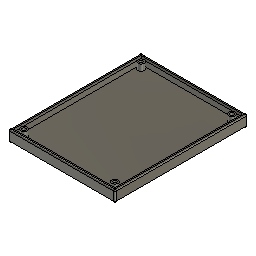
lazyahh_asm (Autodesk Fusion 360 archive; units mm, degrees)
design "ROOM case"
Autodesk Fusion 360 part; units mm, degrees
sketch "Sketch1" plane through (0, 0, 0) normal (0, 0, 1) x (1, 0, 0)
  line L0 (39.5, -50) -> (-39.5, -50)
  line L1 (-39.5, -50) -> (-39.5, 50)
  line L2 (-39.5, 50) -> (39.5, 50)
  line L3 (39.5, 50) -> (39.5, -50)
  line L4 (39.5, -50) -> (-39.5, 50) construction
  line L5 (-39.5, -50) -> (39.5, 50) construction
  line L6 (39.5, 50) -> (36.55, 50)
  line L7 (36.55, 50) -> (36.55, 47.05)
  circle A0 centre (36.55, 47.05) radius 1.35
  circle A1 centre (36.55, 47.05) radius 2.5
  circle A2 centre (36.55, 47.05) radius 2.5
  circle A3 centre (36.55, 47.05) radius 1.35
  line L8 (-39.5, 50) -> (-39.5, 47.05)
  line L9 (-39.5, 47.05) -> (-36.55, 47.05)
  circle A4 centre (36.55, 47.05) radius 1.35
  circle A5 centre (36.55, 47.05) radius 2.5
  circle A6 centre (-36.55, 47.05) radius 1.35
  circle A7 centre (-36.55, 47.05) radius 2.5
  line L10 (0, 0) -> (5, 0)
  circle A8 centre (-36.55, -47.05) radius 2.5
  circle A9 centre (36.55, -47.05) radius 1.35
  circle A10 centre (36.55, -47.05) radius 2.5
  circle A11 centre (-36.55, -47.05) radius 1.35
  line L11 (-42.75, 53.25) -> (42.75, 53.25)
  line L12 (42.75, 53.25) -> (42.75, -53.25)
  line L13 (42.75, -53.25) -> (-42.75, -53.25)
  line L14 (-42.75, -53.25) -> (-42.75, 53.25)
  line L15 (39.75, 50.25) -> (39.75, -50.25)
  line L16 (39.75, -50.25) -> (-39.75, -50.25)
  line L17 (-39.75, -50.25) -> (-39.75, 50.25)
  line L18 (-39.75, 50.25) -> (39.75, 50.25)
  point P0 (36.55, -47.05)
  dimension "d1" = 79
  dimension "d2" = 100
  dimension "d3" = 2.95
  dimension "d4" = 2.95
  dimension "d5" = 2.7
  dimension "d6" = 5
  dimension "d7" = 2.7
  dimension "d8" = 5
  dimension "d9" = 2.95
  dimension "d10" = 2.7
  dimension "d11" = 5
  dimension "d12" = 2.7
  dimension "d13" = 5
  dimension "d14" = -3.25
  dimension "d15" = -0.25
  constraint horizontal L0
  constraint perpendicular L0 L1
  constraint parallel L0 L2
  constraint parallel L1 L3
  constraint coincident L4 L10.start
  constraint coincident L5 L10.start
  constraint coincident L10.start origin
  constraint perpendicular L3 L6
  constraint perpendicular L6 L7
  constraint coincident L7.end A0.centre
  constraint concentric A0 A1
  constraint concentric A2 A3
  constraint perpendicular L2 L8
  constraint perpendicular L1 L9
  constraint coincident L9.end A6.centre
  constraint concentric A6 A7
  constraint horizontal L10
  constraint symmetric A0 L10 A9
  constraint symmetric L7.end L10 P0
  constraint symmetric A5 L10 A10
  constraint symmetric A6 L10 A11
  constraint symmetric A7 L10 A8
  measures "d1" distance of L1.end L2.end
  measures "d2" distance of L0.end L1.end
  measures "d3" distance of L2.end L6.end
  measures "d4" distance of L6.end L7.end
  measures "d5" diameter of A0
  measures "d6" diameter of A1
  measures "d7" diameter of A3
  measures "d8" diameter of A2
  measures "d9" distance of L1.end L8.end
  measures "d10" diameter of A4
  measures "d11" diameter of A5
  measures "d12" diameter of A6
  measures "d13" diameter of A7
extrude "Extrude1" add sketch "Sketch1" along normal blind 4 contours L0 L1 L2 L3 L6 L8 makes body 1
extrude "Extrude2" add sketch "Sketch1" along normal blind 5 separate body contours L11 L12 L13 L14 makes body 2
extrude "Extrude3" add sketch "Sketch1" along normal blind 10 separate body contours A1 A2 A5 | A7 | A8 | A10 makes body 3 at (39.0469, -47.1746, 6.6667) makes body 4 at (39.0376, 47.2989, 6.6667) makes body 5 at (-34.0531, -47.1746, 6.6667) makes body 6 at (-34.0624, 47.2989, 6.6667)
extrude "Extrude4" add 1 faces at (-41.75, -16.75, 5) along direction (0, 0, 1) blind 4 on bodies 2 bodies 2
extrude "Extrude5" add sketch "Sketch1" along normal blind 4 separate body contours A0 A3 A4 | A6 | A9 | A11 makes body 7 at (37.8933, 47.1844, 2.6667) makes body 8 at (-37.8933, -47.1844, 2.6667) makes body 9 at (-35.2067, 47.1844, 2.6667) makes body 10 at (35.2067, -47.1844, 2.6667)
extrude "Extrude6" cut 4 faces at (-34.4426, -47.1742, 10) (38.6574, -47.1742, 10) (38.6523, 47.2413, 10) (-34.4477, 47.2413, 10) along direction (0, 0, -1) blind 1 on bodies 3 4 5 6 bodies 3 4 5 6
fillet "Fillet1" radius 1 12 edges at (42.75, 53.25, 4.5) (0, 53.25, 9) (42.75, 0, 9) (0, 53.25, 0) (42.75, 0, 0) (42.75, -53.25, 4.5) (0, -53.25, 9) (0, -53.25, 0) (-42.75, -53.25, 4.5) (-42.75, 0, 9) (-42.75, 0, 0) (-42.75, 53.25, 4.5) on bodies 2
chamfer "Chamfer1" distance 1 angle 45 4 edges at (0, 50.25, 9) (-39.75, 0, 9) (39.75, 0, 9) (0, -50.25, 9) on bodies 2
